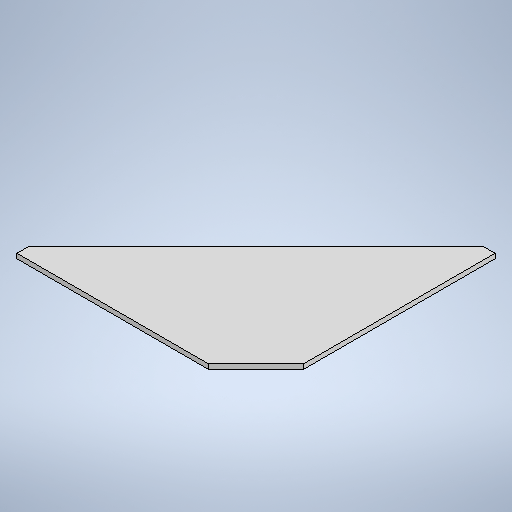
# Autodesk Inventor part: PNS-077 stretch plate
Saved by Autodesk Inventor 2025 (Build 290162010, 162A)
## iProperties
Created: 2025-03-26
Part Number: PNS-077 stretch plate
Material: Stainless Steel
Description: DIE16(5)|\ 90°|corrY -___°|X_____|bom___
Document SubType Name: Sheet Metal
Designer: user
Stock Number: МОО 305 шпангоут борт
Mass: 676.8 g
Surface Area: 449.611 cm^2
Volume: 84.6 cm^3
Density: 8 g/cm^3
Sheet Metal Rule: AISI304 2mm Die16
Sheet Metal Width: 120,208 mm
Sheet Metal Length: 282,843 mm
Sheet Metal Area: 34000,000 mm^2
Appearance: Default
Flat Pattern Width: 12.0208 cm
Flat Pattern Length: 28.2843 cm
Flat Pattern Area: 340 cm^2
Author: admin
Autodesk Inventor part; units mm, degrees
ref_plane "YZ Plane" through (0, 0, 0) normal (1, 0, 0) x (0, 1, 0)
ref_plane "XZ Plane" through (0, 0, 0) normal (0, 1, 0) x (-1, 0, 0)
ref_plane "XY Plane" through (0, 0, 0) normal (0, 0, 1) x (1, 0, 0)
sketch "Sketch1" plane through (0, 0, 0) normal (0, 0, 1) x (1, 0, 0)
  line L0 (0, 0) -> (0, 200)
  line L1 (0, 200) -> (-10, 200)
  line L2 (-10, 200) -> (-200, 10)
  line L3 (-200, 10) -> (-200, 0)
  line L4 (-200, 0) -> (0, 0)
  line L5 (0, 40) -> (-40, 0)
  dimension "d162" = 200
  dimension "d163" = 10
  dimension "d164" = 40
  dimension "d165" = 40
  measures "d162" distance of L0.start L0.end
  measures "d163" distance of L0.end L1.end
  measures "d164" distance of L0.start L5.start
  measures "d165" distance of L0.start L5.end
extrude "Plate5" add sketch "Sketch1" along normal blind 4 contours L5 L4 L3 L2 L1 L0
body "Solid3"
